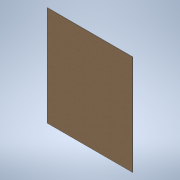
# Autodesk Inventor part: tampa
Saved by Autodesk Inventor 2022 (Build 260153000, 153)
## iProperties
Created: 2022-02-18
Part Number: tampa
Material: MDF - Chapa de fibra de média densidade
Document SubType Name: Modeling
Designer: mathe
Density: 0.8 g/cm^3
Appearance: Papelão - Corrugado
Author: mathe
Autodesk Inventor part; units mm, degrees
ref_plane "YZ Plane" through (0, 0, 0) normal (1, 0, 0) x (0, 1, 0)
ref_plane "XZ Plane" through (0, 0, 0) normal (0, 1, 0) x (-1, 0, 0)
ref_plane "XY Plane" through (0, 0, 0) normal (0, 0, 1) x (1, 0, 0)
sketch "Esboço1" plane through (0, 0, 0) normal (0, 0, 1) x (1, 0, 0)
  line L0 (0, 0) -> (600, 0)
  line L1 (600, 0) -> (600, 700)
  line L2 (600, 700) -> (0, 700)
  line L3 (0, 700) -> (0, 0)
  dimension "d0" = 600
  dimension "d1" = 700
  constraints: 8 end point, 2 parallel, 1 horizontal, 1 perpendicular
  measures "d0" distance of L2.end L1.end
  measures "d1" distance of L1.end L0.end
extrude "Extrusão1" add sketch "Esboço1" along normal blind 3
